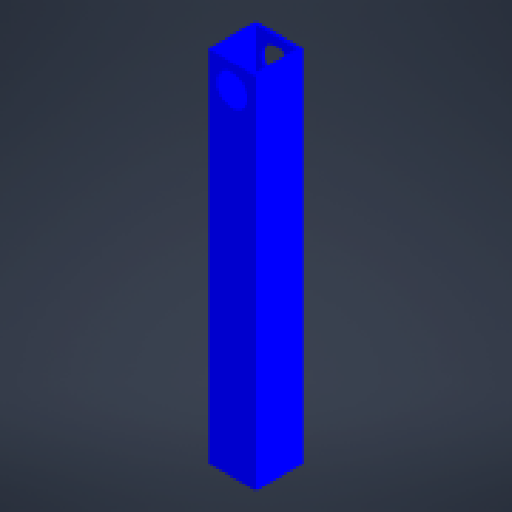
# Autodesk Inventor part: arm
Saved by Autodesk Inventor 2024 (Build 280153000, 153)
## iProperties
Created: 2023-09-26
Part Number: arm
Material: Типовые
Document SubType Name: Modeling
Designer: user
Density: 1 g/cm^3
Appearance: По умолчанию
Author: user
Autodesk Inventor part; units mm, degrees
ref_plane "YZ Plane" through (0, 0, 0) normal (1, 0, 0) x (0, 1, 0)
ref_plane "XZ Plane" through (0, 0, 0) normal (0, 1, 0) x (-1, 0, 0)
ref_plane "XY Plane" through (0, 0, 0) normal (0, 0, 1) x (1, 0, 0)
sketch "Эскиз1" plane through (0, 0, 0) normal (0, 0, 1) x (1, 0, 0)
  line L0 (0, 0) -> (20, 0)
  line L1 (20, 0) -> (20, 20)
  line L2 (20, 20) -> (0, 20)
  line L3 (0, 20) -> (0, 0)
  line L4 (1.5, 18.5) -> (18.5, 18.5)
  line L5 (18.5, 18.5) -> (18.5, 1.5)
  line L6 (18.5, 1.5) -> (1.5, 1.5)
  line L7 (1.5, 1.5) -> (1.5, 18.5)
  dimension "d0" = 1.5
  dimension "d1" = 20
  dimension "d2" = 20
  constraints: 16 end point, 4 parallel, 2 perpendicular, 1 horizontal, 3 other
  measures "d0" horizontal distance of L2.end L4.start
  measures "d1" distance of L1.end L2.end
  measures "d2" distance of L0.end L1.end
extrude "Выдавливание1" add sketch "Эскиз1" along normal blind 150
sketch "Эскиз2" plane through (0, 0, 0) normal (0, -1, 0) x (1, 0, 0)
  circle A0 centre (10, 140) radius 6.5
  line L0 (20, 0) -> (20, 150) projected
  line L1 (0, 150) -> (20, 150) projected
  point P0 (0, 0)
  point P1 (10, 150)
  dimension "d5" = 13
  dimension "d7" = 10
  constraints: 1 centre point, 1 midpoint, 1 vertical alignment
  measures "d5" diameter of A0
  measures "d7" distance from line of L1 A0.centre
extrude "Выдавливание2" cut sketch "Эскиз2" against normal through all
equation "\"d1\" = d2"
